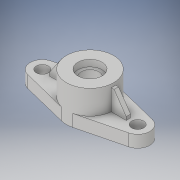
# Autodesk Inventor part: Part2
Saved by Autodesk Inventor 2018 (Build 220112000, 112)
## iProperties
Created: 2017-11-09
Part Number: Part2
Material: Generic
Document SubType Name: Modeling
Designer: kurtis
Density: 1 g/cm^3
Appearance: Default
Author: kurtis
Autodesk Inventor part; units mm, degrees
ref_plane "YZ Plane" through (0, 0, 0) normal (1, 0, 0) x (0, 1, 0)
ref_plane "XZ Plane" through (0, 0, 0) normal (0, 1, 0) x (-1, 0, 0)
ref_plane "XY Plane" through (0, 0, 0) normal (0, 0, 1) x (1, 0, 0)
sketch "Sketch1" plane through (0, 0, 0) normal (0, 0, 1) x (1, 0, 0)
  circle A0 centre (0, 0) radius 10.75
  circle A1 centre (0, 0) radius 5.5
  line L0 (0, 0) -> (21.75, 0) construction
  line L1 (0, 0) -> (-21.75, 0) construction
  circle A2 centre (0, 0) radius 4
  circle A3 centre (21.75, 0) radius 2.75
  circle A4 centre (-21.75, 0) radius 2.75
  arc A5 (-23.0776, 5.3374) -> (-23.0776, -5.3374) centre (-21.75, 0) ccw
  line L2 (-21.75, 0) -> (-21.75, -5.5) construction
  line L3 (-21.75, 0) -> (-21.75, 5.5) construction
  arc A6 (23.0776, -5.3374) -> (23.0776, 5.3374) centre (21.75, 0) ccw
  line L4 (21.75, 0) -> (21.75, -5.5) construction
  line L5 (21.75, 0) -> (21.75, 5.5) construction
  line L6 (-23.0776, 5.3374) -> (-2.5948, 10.4321)
  line L7 (2.5948, 10.4321) -> (23.0776, 5.3374)
  line L8 (23.0776, -5.3374) -> (2.5948, -10.4321)
  line L9 (-23.0776, -5.3374) -> (-2.5948, -10.4321)
  dimension "d0" = 21.5
  dimension "d1" = 11
  dimension "d2" = 21.75
  dimension "d3" = 21.75
  dimension "d4" = 8
  dimension "d5" = 5.5
  dimension "d6" = 5.5
  dimension "d7" = 5.5
  dimension "d8" = 180
  dimension "d9" = 5.5
  dimension "d10" = 180
  constraints: 20 end point, 8 point on circle, 8 tangent, 7 centre point, 7 coincident, 2 horizontal
  measures "d0" diameter of A0
  measures "d1" diameter of A1
  measures "d2" distance of L0.start L0.end
  measures "d3" distance of L0.start L1.end
  measures "d4" diameter of A2
  measures "d5" diameter of A3
  measures "d6" diameter of A4
  measures "d7" radius of A5
  measures "d8" angle of L3 L2
  measures "d9" radius of A6
  measures "d10" angle of L5 L4
extrude "Extrusion1" add sketch "Sketch1" along normal blind 5.5 contours A0 | A0 L7 A6 L8 | A0 L9 A5 L6 | A1
extrude "Extrusion2" add sketch "Sketch1" along normal blind 13.5 contours A0 | A1
extrude "Extrusion3" add sketch "Sketch1" along normal blind 16.5 contours A0
sketch "Sketch2" plane through (0, 0, 5.5) normal (0, 0, 1) x (1, 0, 0)
  line L0 (-17.5, 1) -> (-10.5, 1)
  line L1 (-10.5, 1) -> (-10.5, -1)
  line L2 (-10.5, -1) -> (-17.5, -1)
  line L3 (-17.5, -1) -> (-17.5, 1)
  line L4 (-17.5, 1) -> (-10.5, -1) construction
  line L5 (-10.5, 1) -> (-17.5, -1) construction
  line L6 (10.5, 1) -> (17.5, 1)
  line L7 (17.5, 1) -> (17.5, -1)
  line L8 (17.5, -1) -> (10.5, -1)
  line L9 (10.5, -1) -> (10.5, 1)
  line L10 (10.5, 1) -> (17.5, -1) construction
  line L11 (17.5, 1) -> (10.5, -1) construction
  circle A0 centre (0, 0) radius 10.75 projected
  point P0 (-14, 0)
  point P1 (14, 0)
  dimension "d20" = 7
  dimension "d21" = 7
  dimension "d22" = 2
  dimension "d23" = 0
  dimension "d24" = 2
  dimension "d25" = 10.5
  dimension "d26" = 10.5
  constraints: 24 end point, 4 midpoint, 4 parallel, 2 horizontal, 2 perpendicular, 1 point on line
  measures "d20" distance of L6.start L6.end
  measures "d21" distance of L0.start L0.end
  measures "d22" distance between parallel lines of L8 L6
  measures "d23" vertical distance of point (0, 0) point (14, 0)
  measures "d24" distance between parallel lines of L0 L2
  measures "d25" distance from line of point (0, 0) L9
  measures "d26" distance from line of L1 point (0, 0)
extrude "Extrusion4" cut sketch "Sketch2" along normal blind 9.5 contours L0 A0 L2 L3 | L0 L1 L2 A0 | A0 L8 L9 L6 | L6 L7 L8 A0
sketch "Sketch3" plane through (10.5, -1, 5.5) normal (1, 0, 0) x (0, 0, -1)
  line L0 (-9.5, 2) -> (0, 2) projected
  line L1 (0, 0) -> (-9.5, 0) projected
  line L2 (-9.5, 2) -> (0, 2)
  line L3 (0, 2) -> (0, 0)
  line L4 (0, 0) -> (-9.5, 0)
  line L5 (-9.5, 0) -> (-9.5, 2)
  point P0 (5.5, 1)
  dimension "d29" = 9.5
  dimension "d30" = 2
  constraints: 8 end point, 2 parallel, 1 horizontal, 1 perpendicular
  measures "d29" distance of L1.start L4.end
  measures "d30" distance of L2.end L1.start
sketch "Sketch4" plane through (-10.5, -1, 5.5) normal (-1, 0, 0) x (0, 0, 1)
  line L0 (9.5, 0) -> (0, 0)
  line L1 (0, 0) -> (0, 2)
  line L2 (0, 2) -> (9.5, 2)
  line L3 (9.5, 2) -> (9.5, 0)
  point P0 (-5.5, 1)
  constraints: 8 end point, 2 parallel, 1 horizontal, 1 perpendicular
extrude "Extrusion5" add sketch "Sketch2" along normal blind 1.5 contours L0 A0 L2 L3 | L0 L1 L2 A0 | A0 L8 L9 L6 | L6 L7 L8 A0
extrude "Extrusion6" add sketch "Sketch4" along normal blind 1.5
extrude "Extrusion7" add sketch "Sketch3" along normal blind 1.5
sketch "Sketch5" plane through (10.7034, -1, 5.5) normal (0, -1, 0) x (1, 0, 0)
  line L0 (1.2966, 1.5) -> (1.2966, 9.5) projected
  line L1 (6.7966, 1.5) -> (1.2966, 1.5) projected
  line L2 (1.2966, 9.5) -> (6.7966, 1.5)
  line L3 (6.7966, 1.5) -> (1.2966, 1.5)
  line L4 (1.2966, 1.5) -> (1.2966, 9.5)
  line L5 (-22.7034, 9.5) -> (-22.7034, 1.5) projected
  line L6 (-28.2034, 0) -> (-28.2034, 1.5) projected
  line L7 (-22.7034, 9.5) -> (-28.2034, 1.5)
  line L8 (-22.7034, 1.5) -> (-28.2034, 1.5) projected
  line L9 (-28.2034, 1.5) -> (-22.7034, 1.5)
  line L10 (-22.7034, 1.5) -> (-22.7034, 9.5)
  point P0 (-10.7034, -5.5)
  constraints: 12 end point, 2 collinear, 2 perpendicular
extrude "Extrusion8" add sketch "Sketch5" against normal blind 2
equation "\"d3\" = d2"
equation "\"d6\" = d5"
equation "\"d7\" = d5"
equation "\"d9\" = d5"
body "Solid1"
